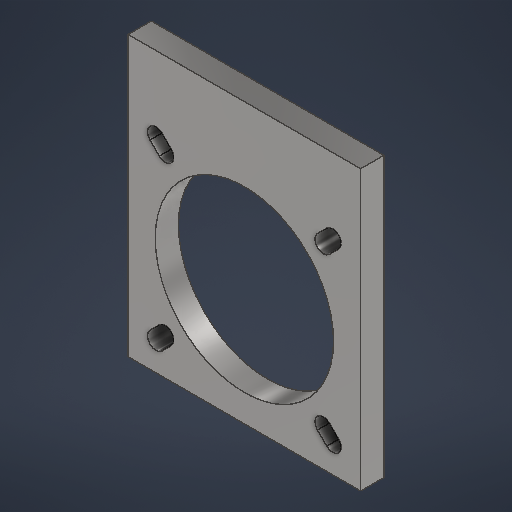
# Autodesk Inventor part: SYSTEM-FLANGE-LOWER
Saved by Autodesk Inventor 2025.3 (Build 293356030, 356C)
## iProperties
Created: 2025-11-27
Part Number: SYSTEM-FLANGE-LOWER
Material: Generic
Document SubType Name: Modeling
Designer: lstk1ng
Density: 1 g/cm^3
Appearance: Semi-Polished
Author: lstk1ng
Autodesk Inventor part; units mm, degrees
ref_plane "YZ Plane" through (0, 0, 0) normal (1, 0, 0) x (0, 1, 0)
ref_plane "XZ Plane" through (0, 0, 0) normal (0, 1, 0) x (-1, 0, 0)
ref_plane "XY Plane" through (0, 0, 0) normal (0, 0, 1) x (1, 0, 0)
sketch "Sketch1" plane through (0, 0, 0) normal (0, 0, 1) x (1, 0, 0)
  line L0 (75, -90) -> (-75, -90)
  line L1 (-75, -90) -> (-75, 90)
  line L2 (-75, 90) -> (75, 90)
  line L3 (75, 90) -> (75, -90)
  line L4 (75, -90) -> (-75, 90) construction
  line L5 (-75, -90) -> (75, 90) construction
  point P0 (0, 0)
  dimension "d0" = 150
  dimension "d1" = 180
  constraints: 12 end point, 2 midpoint, 2 parallel, 1 horizontal, 1 perpendicular
  measures "d0" distance of L1.end L2.end
  measures "d1" distance of L0.end L1.end
extrude "Extrusion1" add sketch "Sketch1" along normal blind 15
sketch "Sketch2" plane through (0, 0, 15) normal (0, 0, 1) x (1, 0, 0)
  line L0 (51, -66) -> (-51, -66) construction
  line L1 (-51, -66) -> (-51, 36) construction
  line L2 (-51, 36) -> (51, 36) construction
  line L3 (51, 36) -> (51, -66) construction
  line L4 (57, -72) -> (-57, -72) construction
  line L5 (-57, -72) -> (-57, 42) construction
  line L6 (-57, 42) -> (57, 42) construction
  line L7 (57, 42) -> (57, -72) construction
  line L8 (-57, 42) -> (-51, 36) construction
  line L9 (-54, 39) -> (-47.1057, 32.1057) construction
  line L10 (-51, 36) -> (-57, 42) construction
  line L11 (-47.1057, 39.8943) -> (-53.1057, 45.8943)
  line L12 (-60.8943, 38.1057) -> (-54.8943, 32.1057)
  arc A0 (-54.8943, 32.1057) -> (-47.1057, 39.8943) centre (-51, 36) ccw
  arc A1 (-53.1057, 45.8943) -> (-60.8943, 38.1057) centre (-57, 42) ccw
  line L13 (51, 36) -> (57, 42) construction
  line L14 (51, -66) -> (57, -72) construction
  line L15 (-51, -66) -> (-57, -72) construction
  line L16 (54, 39) -> (47.1057, 32.1057) construction
  line L17 (54, -69) -> (47.1057, -62.1057) construction
  line L18 (-54, -69) -> (-47.1057, -62.1057) construction
  line L19 (51, 36) -> (57, 42) construction
  line L20 (54.8943, 32.1057) -> (60.8943, 38.1057)
  line L21 (53.1057, 45.8943) -> (47.1057, 39.8943)
  arc A2 (47.1057, 39.8943) -> (54.8943, 32.1057) centre (51, 36) ccw
  arc A3 (60.8943, 38.1057) -> (53.1057, 45.8943) centre (57, 42) ccw
  line L22 (51, -66) -> (57, -72) construction
  line L23 (47.1057, -69.8943) -> (53.1057, -75.8943)
  line L24 (60.8943, -68.1057) -> (54.8943, -62.1057)
  arc A4 (54.8943, -62.1057) -> (47.1057, -69.8943) centre (51, -66) ccw
  arc A5 (53.1057, -75.8943) -> (60.8943, -68.1057) centre (57, -72) ccw
  line L25 (-51, -66) -> (-57, -72) construction
  line L26 (-54.8943, -62.1057) -> (-60.8943, -68.1057)
  line L27 (-53.1057, -75.8943) -> (-47.1057, -69.8943)
  arc A6 (-47.1057, -69.8943) -> (-54.8943, -62.1057) centre (-51, -66) ccw
  arc A7 (-60.8943, -68.1057) -> (-53.1057, -75.8943) centre (-57, -72) ccw
  line L28 (75, 90) -> (-75, 90) construction
  line L29 (-75, 90) -> (75, 90) construction
  line L30 (75, 90) -> (75, 75) construction
  line L31 (75, 75) -> (-75, 75) construction
  line L32 (-75, 75) -> (-75, 90) construction
  line L33 (0, 0) -> (0, -15) construction
  circle A8 centre (0, -15) radius 57.5
  point P0 (54, 39)
  point P1 (54, -69)
  point P2 (-54, -69)
  dimension "d5" = 102
  dimension "d6" = 102
  dimension "d7" = 114
  dimension "d8" = 114
  dimension "d9" = 9.75
  dimension "d12" = 15
  dimension "d13" = 15
  dimension "d14" = 115
  constraints: 74 end point, 16 point on circle, 16 tangent, 10 parallel, 9 centre point, 8 midpoint, 4 collinear, 3 horizontal, 3 perpendicular, 2 point on line, 1 coincident, 1 vertical
  measures "d5" distance of L1.end L2.end
  measures "d6" distance of L0.end L1.end
  measures "d7" distance of L5.end L6.end
  measures "d8" distance of L4.end L5.end
  measures "d9" distance of L9.start L9.end
  measures "d12" distance of L29.end L30.end
  measures "d13" distance of L33.start L33.end
  measures "d14" diameter of A8
extrude "Extrusion2" cut sketch "Sketch2" against normal through all
body "Solid1"
